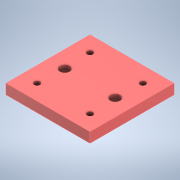
# Autodesk Inventor part: Lagerhalterung
Saved by Autodesk Inventor 2022 (Build 260153000, 153)
## iProperties
Created: 2022-04-21
Part Number: Lagerhalterung
Material: Generisch
Document SubType Name: Modeling
Designer: 123St
Density: 1 g/cm^3
Appearance: Glatt - Rot
Author: 123St
Autodesk Inventor part; units mm, degrees
ref_plane "YZ Plane" through (0, 0, 0) normal (1, 0, 0) x (0, 1, 0)
ref_plane "XZ Plane" through (0, 0, 0) normal (0, 1, 0) x (-1, 0, 0)
ref_plane "XY Plane" through (0, 0, 0) normal (0, 0, 1) x (1, 0, 0)
sketch "Skizze1" plane through (0, 0, 0) normal (0, 1, 0) x (-1, 0, 0)
  line L0 (25, -25) -> (-25, -25)
  line L1 (-25, -25) -> (-25, 25)
  line L2 (-25, 25) -> (25, 25)
  line L3 (25, 25) -> (25, -25)
  line L4 (25, -25) -> (-25, 25) construction
  line L5 (-25, -25) -> (25, 25) construction
  point P0 (0, 0)
  dimension "d0" = 50
  dimension "d1" = 50
  constraints: 12 end point, 2 midpoint, 2 parallel, 1 horizontal, 1 perpendicular
  measures "d0" distance of L0.start L0.end
  measures "d1" distance of L2.end L0.start
extrude "Extrusion1" add sketch "Skizze1" along normal blind 6
sketch "Skizze2" plane through (0, 0, 0) normal (0, -1, 0) x (1, 0, 0)
  circle A0 centre (-15.75, 15.75) radius 4.25
  circle A1 centre (15.75, 15.75) radius 4.25
  circle A2 centre (15.75, -15.75) radius 4.25
  circle A3 centre (-15.75, -15.75) radius 4.25
  line L0 (-35, 0) -> (35, 0) projected
  line L1 (0, 35) -> (0, -35) projected
  point P0 (0, 0)
  dimension "d4" = 31.5
  dimension "d5" = 31.5
  dimension "d6" = 31.5
  dimension "d7" = 31.5
  dimension "d8" = 15.75
  dimension "d9" = 15.75
  dimension "d10" = 15.75
  dimension "d11" = 15.75
  dimension "d12" = 8.5
  dimension "d13" = 8.5
  dimension "d14" = 8.5
  dimension "d15" = 8.5
  constraints: 4 centre point
  measures "d4" distance of A1.centre A0.centre
  measures "d5" distance of A2.centre A3.centre
  measures "d6" distance of A0.centre A3.centre
  measures "d7" distance of A2.centre A1.centre
  measures "d8" distance from line of L0 A3.centre
  measures "d9" distance from line of L0 A2.centre
  measures "d10" distance from line of L1 A2.centre
  measures "d11" distance from line of L1 A1.centre
  measures "d12" diameter of A0
  measures "d13" diameter of A1
  measures "d14" diameter of A3
  measures "d15" diameter of A2
extrude "Extrusion2" add sketch "Skizze2" along normal blind 1
sketch "Skizze3" plane through (-15.75, -1, 15.75) normal (0, -1, 0) x (1, 0, 0)
  circle A0 centre (0, 0) radius 4.25 projected
  circle A1 centre (0, 0) radius 1.75
  circle A2 centre (31.5, 0) radius 4.25 projected
  circle A3 centre (31.5, 0) radius 1.75
  circle A4 centre (31.5, -31.5) radius 4.25 projected
  circle A5 centre (31.5, -31.5) radius 1.75
  circle A6 centre (0, -31.5) radius 4.25 projected
  circle A7 centre (0, -31.5) radius 1.75
  point P0 (15.75, -15.75)
  dimension "d18" = 3.5
  dimension "d19" = 3.5
  dimension "d20" = 3.5
  dimension "d21" = 3.5
  constraints: 4 centre point, 4 coincident
  measures "d18" diameter of A1
  measures "d19" diameter of A3
  measures "d20" diameter of A5
  measures "d21" diameter of A7
extrude "Extrusion3" cut sketch "Skizze3" against normal blind 13 contours A1 | A3 | A5 | A7
sketch "Skizze4" plane through (0, 0, 0) normal (0, -1, 0) x (1, 0, 0)
  circle A0 centre (-15, 0) radius 1.5
  circle A1 centre (15, 0) radius 1.5
  line L0 (0, 35) -> (0, -35) projected
  point P0 (0, 0)
  dimension "d24" = 30
  dimension "d25" = 15
  dimension "d26" = 3
  dimension "d27" = 3
  constraints: 2 centre point
  measures "d24" distance of A1.centre A0.centre
  measures "d25" distance from line of L0 A1.centre
  measures "d26" diameter of A0
  measures "d27" diameter of A1
extrude "Extrusion4" cut sketch "Skizze4" against normal blind 13
sketch "Skizze7" plane through (0, 6, 0) normal (0, 1, 0) x (1, 0, 0)
  circle A0 centre (15, 0) radius 1.5 projected
  circle A1 centre (15, 0) radius 3
  circle A2 centre (-15, 0) radius 1.5 projected
  circle A3 centre (-15, 0) radius 3
  point P0 (0, 0)
  dimension "d39" = 6
  dimension "d40" = 6
  constraints: 2 centre point, 2 coincident
  measures "d39" diameter of A1
  measures "d40" diameter of A3
extrude "Extrusion5" cut sketch "Skizze7" against normal blind 4 contours A0 | A1 | A2 | A3
chamfer "Fase1" distance 1 angle 45 2 edges at (12, 2, 0) (-18, 2, 0)
equation "\"d8\" = 0.5 * d6"
equation "\"d9\" = 0.5 * d7"
equation "\"d10\" = 0.5 * d5"
equation "\"d11\" = 0.5 * d4"
equation "\"d25\" = 0.5 * d24"
